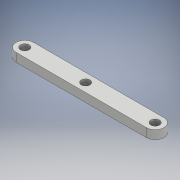
# Autodesk Inventor part: panto_linkageC
Saved by Autodesk Inventor 2017 (Build 210142000, 142)
## iProperties
Created: 2018-01-12
Part Number: panto_linkageC
Material: Generic
Document SubType Name: Modeling
Designer: Nic
Density: 1 g/cm^3
Appearance: Default
Author: Nic
Autodesk Inventor part; units mm, degrees
ref_plane "YZ Plane" through (0, 0, 0) normal (1, 0, 0) x (0, 1, 0)
ref_plane "XZ Plane" through (0, 0, 0) normal (0, 1, 0) x (-1, 0, 0)
ref_plane "XY Plane" through (0, 0, 0) normal (0, 0, 1) x (1, 0, 0)
sketch "Sketch1" plane through (0, 0, 0) normal (0, 0, 1) x (1, 0, 0)
  circle A0 centre (0, 0) radius 1
  circle A1 centre (-14, 0) radius 1
  line L0 (-14, 2) -> (16, 2)
  line L1 (16, -2) -> (-14, -2)
  arc A2 (-14, 2) -> (-14, -2) centre (-14, 0) ccw
  circle A3 centre (16, 0) radius 1
  arc A4 (16, -2) -> (16, 2) centre (16, 0) ccw
  dimension "d0" = 2
  dimension "d1" = 14
  dimension "d5" = 16
  dimension "d6" = 2
  constraints: 5 centre point, 4 end point, 4 point on circle, 4 tangent, 3 vertical alignment, 2 equal radius, 2 horizontal alignment, 1 coincident, 1 concentric, 1 horizontal, 1 parallel
  measures "d0" diameter of A0
  measures "d1" distance of point (0, 0) A1.centre
  measures "d5" distance of A3.centre point (0, 0)
  measures "d6" radius of A4
extrude "Extrusion1" add sketch "Sketch1" along normal blind 2
body "Solid1"
